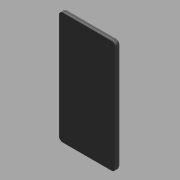
# Autodesk Inventor part: END CAP 3060
Saved by Autodesk Inventor 2016 (Build 200138000, 138)
## iProperties
Created: 2023-12-03
Part Number: END CAP 3060
Material: Generic
Document SubType Name: Modeling
Designer: Riskinova Oktavia
Density: 1 g/cm^3
Appearance: Default
Author: Riskinova Oktavia
Autodesk Inventor part; units mm, degrees
ref_plane "YZ Plane" through (0, 0, 0) normal (1, 0, 0) x (0, 1, 0)
ref_plane "XZ Plane" through (0, 0, 0) normal (0, 1, 0) x (-1, 0, 0)
ref_plane "XY Plane" through (0, 0, 0) normal (0, 0, 1) x (1, 0, 0)
sketch "Sketch1" plane through (0, 0, 0) normal (0, 1, 0) x (-1, 0, 0)
  line L0 (-13, 30) -> (13, 30)
  line L1 (15, 28) -> (15, -28)
  line L2 (13, -30) -> (-13, -30)
  line L3 (-15, -28) -> (-15, 28)
  line L4 (-15, 30) -> (15, -30) construction
  line L5 (15, 30) -> (-15, -30) construction
  arc A0 (15, 28) -> (13, 30) centre (13, 28) ccw
  arc A1 (13, -30) -> (15, -28) centre (13, -28) ccw
  arc A2 (-15, -28) -> (-13, -30) centre (-13, -28) ccw
  arc A3 (-13, 30) -> (-15, 28) centre (-13, 28) ccw
  point P0 (0, 0)
  dimension "d0" = 60
  dimension "d1" = 30
  dimension "d4" = 2
  dimension "d5" = 2
  constraints: 12 end point, 8 point on circle, 8 point on line, 8 tangent, 4 centre point, 2 equal radius, 2 midpoint, 2 parallel, 1 horizontal, 1 perpendicular
  measures "d0" distance of L5.start L4.end
  measures "d1" distance of L4.end L5.end
  measures "d4" radius of A0
  measures "d5" radius of A3
extrude "Extrusion1" add sketch "Sketch1" along normal mid plane 3
fillet "Fillet1" radius 1.5 8 edges at (14.4142, 1.5, -29.4142) (0, 1.5, -30) (-14.4142, 1.5, -29.4142) (-15, 1.5, 0) (-14.4142, 1.5, 29.4142) (0, 1.5, 30) (14.4142, 1.5, 29.4142) (15, 1.5, 0)
body "Solid1"
